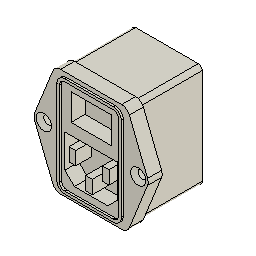
IEC Power and switch 15A v0 (Autodesk Fusion 360 design; units mm, degrees)
Autodesk Fusion 360 part; units mm, degrees
sketch "Sketch1" plane through (0, 0, 0) normal (0, 1, 0) x (1, 0, 0)
  line L0 (-17.9959, 0) -> (17.9959, 0) construction
  line L1 (13.8049, 20.5994) -> (-13.8049, 20.5994)
  line L2 (-13.8049, 20.5994) -> (-13.8049, -20.5994)
  line L3 (-13.8049, -20.5994) -> (13.8049, -20.5994)
  line L4 (13.8049, -20.5994) -> (13.8049, 20.5994)
  line L5 (13.8049, 20.5994) -> (-13.8049, -20.5994) construction
  line L6 (-13.8049, 20.5994) -> (13.8049, -20.5994) construction
  line L7 (-13.8049, -20.5994) -> (-22.0345, 0)
  line L8 (-22.0345, 0) -> (-13.8049, 20.5994)
  line L9 (13.8049, -20.5994) -> (22.0345, 0)
  line L10 (22.0345, 0) -> (13.8049, 20.5994)
  line L11 (-7.62, -15.24) -> (7.62, -15.24)
  line L12 (7.62, -15.24) -> (7.62, -5.08)
  line L13 (7.62, -5.08) -> (-7.62, -5.08)
  line L14 (-7.62, -5.08) -> (-7.62, -15.24)
  line L15 (0, -15.24) -> (0, 0) construction
  line L16 (-9.9798, -0.762) -> (9.9798, -0.762)
  line L17 (9.9798, -0.762) -> (9.9798, 11.8642)
  line L18 (-9.9798, 11.8642) -> (-9.9798, -0.762)
  line L19 (-9.9798, 11.8642) -> (-6.35, 15.494)
  line L20 (6.35, 15.494) -> (9.9798, 11.8642)
  line L21 (9.2329, 18.0594) -> (-9.2329, 18.0594)
  line L22 (-11.2649, 16.0274) -> (-11.2649, -16.0274)
  line L23 (-9.2329, -18.0594) -> (9.2329, -18.0594)
  line L24 (11.2649, -16.0274) -> (11.2649, 16.0274)
  line L25 (0, 17.78) -> (0, 0) construction
  line L26 (-1.27, 8.89) -> (1.27, 8.89)
  line L27 (1.27, 8.89) -> (1.27, 13.97)
  line L28 (1.27, 13.97) -> (-1.27, 13.97)
  line L29 (-1.27, 13.97) -> (-1.27, 8.89)
  line L30 (-5.08, 2.54) -> (-7.62, 2.54)
  line L31 (-7.62, 2.54) -> (-7.62, 7.62)
  line L32 (-7.62, 7.62) -> (-5.08, 7.62)
  line L33 (-5.08, 7.62) -> (-5.08, 2.54)
  line L34 (5.08, 2.54) -> (7.62, 2.54)
  line L35 (7.62, 2.54) -> (7.62, 7.62)
  line L36 (7.62, 7.62) -> (5.08, 7.62)
  line L37 (5.08, 7.62) -> (5.08, 2.54)
  line L38 (-6.35, 15.494) -> (6.35, 15.494)
  line L39 (0, 15.494) -> (0, 0) construction
  arc A0 (-11.2649, -16.0274) -> (-9.2329, -18.0594) centre (-9.2329, -16.0274) ccw
  arc A1 (9.2329, -18.0594) -> (11.2649, -16.0274) centre (9.2329, -16.0274) ccw
  arc A2 (11.2649, 16.0274) -> (9.2329, 18.0594) centre (9.2329, 16.0274) ccw
  arc A3 (-9.2329, 18.0594) -> (-11.2649, 16.0274) centre (-9.2329, 16.0274) ccw
  line L40 (12.2809, -16.0274) -> (12.2809, 16.0274)
  arc A4 (12.2809, 16.0274) -> (9.2329, 19.0754) centre (9.2329, 16.0274) ccw
  line L41 (9.2329, 19.0754) -> (-9.2329, 19.0754)
  arc A5 (-9.2329, 19.0754) -> (-12.2809, 16.0274) centre (-9.2329, 16.0274) ccw
  line L42 (-12.2809, 16.0274) -> (-12.2809, -16.0274)
  arc A6 (-12.2809, -16.0274) -> (-9.2329, -19.0754) centre (-9.2329, -16.0274) ccw
  line L43 (-9.2329, -19.0754) -> (9.2329, -19.0754)
  arc A7 (9.2329, -19.0754) -> (12.2809, -16.0274) centre (9.2329, -16.0274) ccw
  point P0 (-31.8996, 0)
  dimension "d2" = 27.6098
  dimension "d3" = 41.1988
  dimension "d5" = 35.9918
  dimension "d6" = 44.069
  dimension "d7" = 15.24
  dimension "d8" = 10.16
  dimension "d11" = 2.54
  dimension "d12" = 5.08
  dimension "d13" = 5.08
  dimension "d14" = 5.08
  dimension "d15" = 8.89
  dimension "d16" = 135
  dimension "d17" = 16.256
  dimension "d18" = 1.27
  dimension "d19" = 0.762
  dimension "d20" = 19.9595
  dimension "d21" = 12.7
  dimension "d22" = 15.24
  dimension "d32" = 2.032
  dimension "d33" = 1.016
  constraint horizontal L0
  constraint midpoint L15.end L0
  constraint horizontal L1
  constraint perpendicular L1 L2
  constraint parallel L1 L3
  constraint parallel L2 L4
  constraint coincident L5 L15.end
  constraint coincident L6 L15.end
  constraint coincident L15.end L25.end
  constraint parallel L8 L9
  constraint parallel L7 L10
  constraint horizontal L11
  constraint vertical L12
  constraint horizontal L13
  constraint vertical L14
  constraint midpoint L11 L15.start
  constraint vertical L15
  constraint horizontal L16
  constraint vertical L17
  constraint vertical L18
  constraint equal L19 L20
  constraint horizontal L18.start L17.end
  constraint vertical L25
  constraint horizontal L26
  constraint vertical L27
  constraint horizontal L28
  constraint vertical L29
  constraint horizontal L30
  constraint vertical L31
  constraint horizontal L32
  constraint vertical L33
  constraint horizontal L34
  constraint vertical L35
  constraint horizontal L36
  constraint vertical L37
  constraint equal L27 L35
  constraint equal L27 L33
  constraint equal L26 L30
  constraint equal L26 L34
  constraint midpoint L25 L26
  constraint horizontal L38
  constraint collinear L32 L36
  constraint midpoint L38 L39.start
  constraint vertical L39
  constraint horizontal L7.end L9.end
  constraint tangent L23 A0
  constraint tangent L22 A0
  constraint tangent L23 A1
  constraint tangent L24 A1
  constraint equal A0 A1
  constraint tangent L24 A2
  constraint tangent L21 A2
  constraint equal A0 A2
  constraint tangent L21 A3
  constraint tangent L22 A3
  constraint equal A0 A3
  measures "d2" distance of L2.end L3.end
  measures "d3" distance of L1.end L2.end
  measures "d5" distance of L0.start L0.end
  measures "d6" distance of L7.end L9.end
  measures "d7" distance of L11.start L11.end
  measures "d8" distance of L11.end L12.end
  measures "d11" distance of L30.start L30.end
  measures "d12" distance of L30.end L31.end
  measures "d13" horizontal distance of L15.end L30.start
  measures "d14" horizontal distance of L15.end L34.start
  measures "d15" vertical distance of L15.end L26.end
  measures "d16" angle of L20 L38
  measures "d17" distance of L16 L38
  measures "d18" vertical distance of L26.end L36.end
  measures "d19" distance of L0 L16
  measures "d20" distance of L17 L18
  measures "d21" distance of L19.end L20.start
  measures "d22" vertical distance of L15.end L11.end
  measures "d32" radius of A0
extrude "Extrude1" add sketch "Sketch1" along normal blind 5.334 contours L1 L2 L3 L4 | L4 L9 L10 | L2 L7 L8 | L21 L22 L23 L24 A0 A1 A2 A3 | L26 L27 L28 L29 | L30 L31 L32 L33 | L34 L35 L36 L37 | L40 A4 L41 A5 L42 A6 L43 A7 makes body 1 at (-1.27, 1.778, -12.2767) makes body 2 at (5.08, 1.778, -5.9267) makes body 3 at (-7.62, 1.778, -4.2333) makes body 4 at (14.4865, 0, 8.5598)
hole "Hole1" at (-17.9959, 0, 0) at (17.9959, 0, 0) direction (0, 1, 0) diameter 3.175 depth 12.7 tip angle 118 countersink diameter 5.842 countersink angle 82 bodies 4
fillet "Fillet1" radius 3.175 6 edges at (-22.0345, 2.667, 0) (-13.8049, 2.667, 20.5994) (13.8049, 2.667, 20.5994) (22.0345, 2.667, 0) (13.8049, 2.667, -20.5994) (-13.8049, 2.667, -20.5994) on bodies 4
extrude "Extrude2" add sketch "Sketch1" against normal blind 0.762 contours L26 L27 L28 L29 | L30 L31 L32 L33 | L34 L35 L36 L37 | L40 A4 L41 A5 L42 A6 L43 A7 bodies 1 2 3 4
sketch "Sketch2" plane through (0, 5.334, 0) normal (0, 1, 0) x (-1, 0, 0)
  arc A0 (11.6543, -20.5994) -> (14.6028, -18.6023) centre (11.6543, -17.4244) ccw
  line L0 (14.6028, -18.6023) -> (21.5639, -1.1779)
  arc A1 (21.5639, -1.1779) -> (21.5639, 1.1779) centre (18.6155, 0) ccw
  line L1 (21.5639, 1.1779) -> (14.6028, 18.6023)
  arc A2 (14.6028, 18.6023) -> (11.6543, 20.5994) centre (11.6543, 17.4244) ccw
  line L2 (11.6543, 20.5994) -> (-11.6543, 20.5994)
  arc A3 (-11.6543, 20.5994) -> (-14.6028, 18.6023) centre (-11.6543, 17.4244) ccw
  line L3 (-14.6028, 18.6023) -> (-21.5639, 1.1779)
  arc A4 (-21.5639, 1.1779) -> (-21.5639, -1.1779) centre (-18.6155, 0) ccw
  line L4 (-21.5639, -1.1779) -> (-14.6028, -18.6023)
  arc A5 (-14.6028, -18.6023) -> (-11.6543, -20.5994) centre (-11.6543, -17.4244) ccw
  line L5 (-11.6543, -20.5994) -> (11.6543, -20.5994)
  circle A6 centre (17.9959, 0) radius 1.5875
  circle A7 centre (-17.9959, 0) radius 1.5875
  line L6 (9.9798, 0.762) -> (9.9798, -11.8642)
  line L7 (9.9798, -11.8642) -> (6.35, -15.494)
  line L8 (6.35, -15.494) -> (-6.35, -15.494)
  line L9 (-6.35, -15.494) -> (-9.9798, -11.8642)
  line L10 (-9.9798, -11.8642) -> (-9.9798, 0.762)
  line L11 (-9.9798, 0.762) -> (9.9798, 0.762)
  line L12 (7.62, 15.24) -> (7.62, 5.08)
  line L13 (7.62, 5.08) -> (-7.62, 5.08)
  line L14 (-7.62, 5.08) -> (-7.62, 15.24)
  line L15 (-7.62, 15.24) -> (7.62, 15.24)
  line L16 (11.938, -19.812) -> (-11.938, -19.812)
  line L17 (-13.462, -18.288) -> (-13.462, 18.288)
  line L18 (-11.938, 19.812) -> (11.938, 19.812)
  line L19 (13.462, 18.288) -> (13.462, -18.288)
  line L20 (13.462, -19.812) -> (-13.462, 19.812) construction
  line L21 (-13.462, -19.812) -> (13.462, 19.812) construction
  arc A8 (-11.938, 19.812) -> (-13.462, 18.288) centre (-11.938, 18.288) ccw
  arc A9 (13.462, 18.288) -> (11.938, 19.812) centre (11.938, 18.288) ccw
  arc A10 (11.938, -19.812) -> (13.462, -18.288) centre (11.938, -18.288) ccw
  arc A11 (-13.462, -18.288) -> (-11.938, -19.812) centre (-11.938, -18.288) ccw
  dimension "d36" = 26.924
  dimension "d37" = 39.624
  dimension "d38" = 1.524
  constraint horizontal L16
  constraint perpendicular L16 L17
  constraint parallel L16 L18
  constraint parallel L17 L19
  constraint coincident L20 origin
  constraint coincident L21 origin
  constraint coincident L20.end L18
  constraint coincident L20.end L17
  constraint tangent L18 A8
  constraint tangent L17 A8
  constraint coincident L21.end L18
  constraint coincident L21.end L19
  constraint tangent L18 A9
  constraint tangent L19 A9
  constraint equal A8 A9
  constraint coincident L20.start L19
  constraint coincident L20.start L16
  constraint tangent L19 A10
  constraint tangent L16 A10
  constraint equal A8 A10
  constraint coincident L21.start L17
  constraint coincident L21.start L16
  constraint tangent L17 A11
  constraint tangent L16 A11
  constraint equal A8 A11
  measures "d36" distance of L20.end L21.end
  measures "d37" distance of L21.start L20.end
  measures "d38" radius of A8
extrude "Extrude3" add sketch "Sketch2" along normal blind 23.622 contours L6 L7 L8 L9 L10 L11 | L12 L13 L14 L15 | L16 L17 L18 L19 A8 A9 A10 A11 bodies 1 2 3 4
